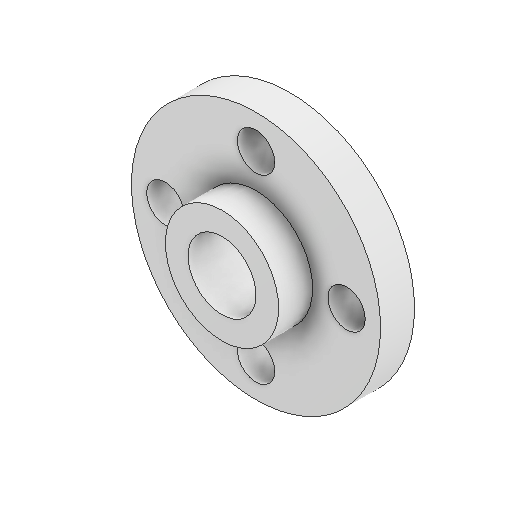
# Autodesk Inventor part: Acople
Saved by Autodesk Inventor 2025.3 (Build 293356000, 356)
## iProperties
Created: 2025-10-28
Part Number: Acople
Material: ABS Plastic
Document SubType Name: Modeling
Designer: Gabriel Bojaca
Density: 1.06 g/cm^3
Appearance: Smooth - White
Author: Gabriel Bojaca
Autodesk Inventor part; units mm, degrees
ref_plane "YZ Plane" through (0, 0, 0) normal (1, 0, 0) x (0, 1, 0)
ref_plane "XZ Plane" through (0, 0, 0) normal (0, 1, 0) x (-1, 0, 0)
ref_plane "XY Plane" through (0, 0, 0) normal (0, 0, 1) x (1, 0, 0)
sketch "Sketch1" plane through (0, 0, 0) normal (0, 0, 1) x (1, 0, 0)
  circle A0 centre (0, 0) radius 11
  circle A1 centre (0, 8) radius 1.65
  line L0 (-3.4226, 0) -> (4.8397, 0) construction
  line L1 (0, 0) -> (0, 2.4255) construction
  circle A2 centre (8, 0) radius 1.65
  circle A3 centre (0, -8) radius 1.65
  circle A4 centre (-8, 0) radius 1.65
  dimension "d0" = 22
  dimension "d1" = 8
  dimension "d2" = 3.3
  dimension "d3" = 8
  dimension "d4" = 3.3
  constraints: 5 centre point, 4 end point, 2 symmetric about line, 1 coincident, 1 horizontal, 1 vertical, 2 other
  measures "d0" diameter of A0
  measures "d1" distance of point (0, 0) A1.centre
  measures "d2" diameter of A2
  measures "d3" distance of A2.centre point (0, 0)
  measures "d4" diameter of A1
extrude "Extrusion1" add sketch "Sketch1" along normal blind 3
sketch "Sketch2" plane through (0, 0, 3) normal (0, 0, 1) x (1, 0, 0)
  circle A0 centre (0, 0) radius 5
  dimension "d7" = 10
  constraints: 1 centre point, 1 coincident
  measures "d7" diameter of A0
extrude "Extrusion2" add sketch "Sketch2" along normal blind 3
sketch "Sketch3" plane through (0, 0, 6) normal (0, 0, 1) x (1, 0, 0)
  circle A0 centre (0, 0) radius 3
  dimension "d10" = 6
  constraints: 1 centre point, 1 coincident
  measures "d10" diameter of A0
extrude "Extrusion3" cut sketch "Sketch3" against normal through all
equation "\"d3\" = d1"
equation "\"d4\" = d2"
body "Solid1"
